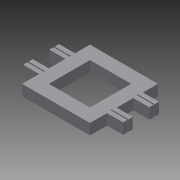
# Autodesk Inventor part: printed carriage v2
Saved by Autodesk Inventor 2014 SP1 (Build 180222100, 222)
## iProperties
Created: 2014-10-27
Part Number: printed carriage v2
Material: Generic
Document SubType Name: Modeling
Designer: dave
Density: 1 g/cm^3
Appearance: Default
Author: dave
Autodesk Inventor part; units mm, degrees
ref_plane "YZ Plane" through (0, 0, 0) normal (1, 0, 0) x (0, 1, 0)
ref_plane "XZ Plane" through (0, 0, 0) normal (0, 1, 0) x (-1, 0, 0)
ref_plane "XY Plane" through (0, 0, 0) normal (0, 0, 1) x (1, 0, 0)
sketch "Sketch1" plane through (0, 0, 0) normal (0, 0, 1) x (1, 0, 0)
  line L0 (0, 0) -> (63.5, 0)
  line L1 (63.5, 63.5) -> (0, 63.5)
  line L2 (0, 2) -> (0, 16) construction
  line L3 (0, 20.5) -> (-60, 20.5) construction
  line L4 (-60, 20.5) -> (152, 20.5) construction
  line L5 (0, 45) -> (-57, 45) construction
  line L6 (-57, 45) -> (114, 45) construction
  line L7 (0, 16) -> (-15, 16)
  line L8 (-15, 25) -> (0, 25)
  line L9 (0, 16) -> (0, 0)
  line L10 (0, 0) -> (12.5, 0) construction
  line L11 (12.5, 0) -> (12.5, 12.5) construction
  line L12 (12.5, 12.5) -> (18.4945, 12.5) construction
  line L13 (63.5, 63.5) -> (63.5, 51) construction
  line L14 (63.5, 51) -> (51, 51) construction
  line L15 (51, 51) -> (12.5, 51)
  line L16 (12.5, 51) -> (12.5, 12.5)
  line L17 (12.5, 12.5) -> (51, 12.5)
  line L18 (51, 12.5) -> (51, 51)
  line L19 (0, 40.5) -> (-15, 40.5)
  line L20 (-15, 49.5) -> (0, 49.5)
  line L21 (0.2886, 45.1642) -> (0.1212, 45.6242)
  line L22 (0.1212, 45.6242) -> (-0.6388, 45.6242)
  line L23 (-0.6388, 45.6242) -> (-0.8062, 45.1642)
  line L24 (-0.8062, 45.1642) -> (-1.7414, 45.1642)
  line L25 (-1.7414, 45.1642) -> (-1.9088, 45.6242)
  line L26 (-1.9088, 45.6242) -> (-2.6688, 45.6242)
  line L27 (-2.6688, 45.6242) -> (-2.8362, 45.1642)
  line L28 (-2.8362, 45.1642) -> (-3.7714, 45.1642)
  line L29 (-3.7714, 45.1642) -> (-3.9388, 45.6242)
  line L30 (-3.9388, 45.6242) -> (-4.6988, 45.6242)
  line L31 (-4.6988, 45.6242) -> (-4.8662, 45.1642)
  line L32 (-4.8662, 45.1642) -> (-5.8014, 45.1642)
  line L33 (-5.8014, 45.1642) -> (-5.9688, 45.6242)
  line L34 (-5.9688, 45.6242) -> (-6.7288, 45.6242)
  line L35 (-6.7288, 45.6242) -> (-6.8962, 45.1642)
  line L36 (-6.8962, 45.1642) -> (-7.8314, 45.1642)
  line L37 (-7.8314, 45.1642) -> (-7.9988, 45.6242)
  line L38 (-7.9988, 45.6242) -> (-8.7588, 45.6242)
  line L39 (-8.7588, 45.6242) -> (-8.9262, 45.1642)
  line L40 (-8.9262, 45.1642) -> (-9.8614, 45.1642)
  line L41 (-9.8614, 45.1642) -> (-10.0288, 45.6242)
  line L42 (-10.0288, 45.6242) -> (-10.7888, 45.6242)
  line L43 (-10.7888, 45.6242) -> (-10.9562, 45.1642)
  line L44 (-10.9562, 45.1642) -> (-11.8914, 45.1642)
  line L45 (-11.8914, 45.1642) -> (-12.0588, 45.6242)
  line L46 (-12.0588, 45.6242) -> (-12.8188, 45.6242)
  line L47 (-12.8188, 45.6242) -> (-12.9862, 45.1642)
  line L48 (-12.9862, 45.1642) -> (-13.9214, 45.1642)
  line L49 (-13.9214, 45.1642) -> (-14.0888, 45.6242)
  line L50 (-14.0888, 45.6242) -> (-14.8488, 45.6242)
  line L51 (-14.8488, 45.6242) -> (-15, 45.2088)
  line L52 (-15.0162, 44.4142) -> (0.2886, 44.4142)
  line L53 (0.3194, 20.653) -> (0.152, 21.113)
  line L54 (0.152, 21.113) -> (-0.608, 21.113)
  line L55 (-0.608, 21.113) -> (-0.7755, 20.653)
  line L56 (-0.7755, 20.653) -> (-1.7106, 20.653)
  line L57 (-1.7106, 20.653) -> (-1.878, 21.113)
  line L58 (-1.878, 21.113) -> (-2.638, 21.113)
  line L59 (-2.638, 21.113) -> (-2.8055, 20.653)
  line L60 (-2.8055, 20.653) -> (-3.7406, 20.653)
  line L61 (-3.7406, 20.653) -> (-3.908, 21.113)
  line L62 (-3.908, 21.113) -> (-4.668, 21.113)
  line L63 (-4.668, 21.113) -> (-4.8355, 20.653)
  line L64 (-4.8355, 20.653) -> (-5.7706, 20.653)
  line L65 (-5.7706, 20.653) -> (-5.938, 21.113)
  line L66 (-5.938, 21.113) -> (-6.698, 21.113)
  line L67 (-6.698, 21.113) -> (-6.8655, 20.653)
  line L68 (-6.8655, 20.653) -> (-7.8006, 20.653)
  line L69 (-7.8006, 20.653) -> (-7.968, 21.113)
  line L70 (-7.968, 21.113) -> (-8.728, 21.113)
  line L71 (-8.728, 21.113) -> (-8.8955, 20.653)
  line L72 (-8.8955, 20.653) -> (-9.8306, 20.653)
  line L73 (-9.8306, 20.653) -> (-9.998, 21.113)
  line L74 (-9.998, 21.113) -> (-10.758, 21.113)
  line L75 (-10.758, 21.113) -> (-10.9255, 20.653)
  line L76 (-10.9255, 20.653) -> (-11.8606, 20.653)
  line L77 (-11.8606, 20.653) -> (-12.028, 21.113)
  line L78 (-12.028, 21.113) -> (-12.788, 21.113)
  line L79 (-12.788, 21.113) -> (-12.9555, 20.653)
  line L80 (-12.9555, 20.653) -> (-13.8906, 20.653)
  line L81 (-13.8906, 20.653) -> (-14.058, 21.113)
  line L82 (-14.058, 21.113) -> (-14.8177, 21.113)
  line L83 (-14.8177, 21.113) -> (-15, 20.6122)
  line L84 (-15, 19.903) -> (0.3194, 19.903)
  line L85 (0, 63.5) -> (0, 49.5) construction
  line L86 (0, 63.5) -> (0, 49.5)
  line L87 (0, 40.5) -> (0, 25)
  line L88 (0.2886, 45.1642) -> (0.2886, 44.4142)
  line L89 (-15, 40.5) -> (-15, 44.4142)
  line L90 (-15, 45.2088) -> (-15, 49.5)
  line L91 (0.3194, 20.653) -> (0.3194, 19.903)
  line L92 (-15, 16) -> (-15, 19.903)
  line L93 (-15, 20.6122) -> (-15, 25)
  line L94 (63.5, 40.5) -> (78.5, 40.5)
  line L95 (78.5, 49.5) -> (63.5, 49.5)
  line L96 (63.5, 16) -> (78.5, 16)
  line L97 (63.5, 25) -> (78.5, 25)
  line L98 (78.5, 20.8487) -> (77.9976, 20.8487)
  line L99 (77.9976, 20.8487) -> (77.8302, 21.3087)
  line L100 (77.8302, 21.3087) -> (77.0702, 21.3087)
  line L101 (77.0702, 21.3087) -> (76.9027, 20.8487)
  line L102 (76.9027, 20.8487) -> (75.9676, 20.8487)
  line L103 (75.9676, 20.8487) -> (75.8002, 21.3087)
  line L104 (75.8002, 21.3087) -> (75.0402, 21.3087)
  line L105 (75.0402, 21.3087) -> (74.8727, 20.8487)
  line L106 (74.8727, 20.8487) -> (73.9376, 20.8487)
  line L107 (73.9376, 20.8487) -> (73.7702, 21.3087)
  line L108 (73.7702, 21.3087) -> (73.0102, 21.3087)
  line L109 (73.0102, 21.3087) -> (72.8427, 20.8487)
  line L110 (72.8427, 20.8487) -> (71.9076, 20.8487)
  line L111 (71.9076, 20.8487) -> (71.7402, 21.3087)
  line L112 (71.7402, 21.3087) -> (70.9802, 21.3087)
  line L113 (70.9802, 21.3087) -> (70.8127, 20.8487)
  line L114 (70.8127, 20.8487) -> (69.8776, 20.8487)
  line L115 (69.8776, 20.8487) -> (69.7102, 21.3087)
  line L116 (69.7102, 21.3087) -> (68.9502, 21.3087)
  line L117 (68.9502, 21.3087) -> (68.7827, 20.8487)
  line L118 (68.7827, 20.8487) -> (67.8476, 20.8487)
  line L119 (67.8476, 20.8487) -> (67.6802, 21.3087)
  line L120 (67.6802, 21.3087) -> (66.9202, 21.3087)
  line L121 (66.9202, 21.3087) -> (66.7527, 20.8487)
  line L122 (66.7527, 20.8487) -> (65.8176, 20.8487)
  line L123 (65.8176, 20.8487) -> (65.6502, 21.3087)
  line L124 (65.6502, 21.3087) -> (64.8902, 21.3087)
  line L125 (64.8902, 21.3087) -> (64.7227, 20.8487)
  line L126 (64.7227, 20.8487) -> (63.7876, 20.8487)
  line L127 (63.7876, 20.8487) -> (63.6202, 21.3087)
  line L128 (63.6202, 21.3087) -> (62.8602, 21.3087)
  line L129 (62.8602, 21.3087) -> (62.6927, 20.8487)
  line L130 (62.6927, 20.8487) -> (62.6927, 20.0987)
  line L131 (62.6927, 20.0987) -> (78.5, 20.0987)
  line L132 (78.5, 45.3158) -> (77.9976, 45.3158)
  line L133 (77.9976, 45.3158) -> (77.8302, 45.7758)
  line L134 (77.8302, 45.7758) -> (77.0702, 45.7758)
  line L135 (77.0702, 45.7758) -> (76.9027, 45.3158)
  line L136 (76.9027, 45.3158) -> (75.9676, 45.3158)
  line L137 (75.9676, 45.3158) -> (75.8002, 45.7758)
  line L138 (75.8002, 45.7758) -> (75.0402, 45.7758)
  line L139 (75.0402, 45.7758) -> (74.8727, 45.3158)
  line L140 (74.8727, 45.3158) -> (73.9376, 45.3158)
  line L141 (73.9376, 45.3158) -> (73.7702, 45.7758)
  line L142 (73.7702, 45.7758) -> (73.0102, 45.7758)
  line L143 (73.0102, 45.7758) -> (72.8427, 45.3158)
  line L144 (72.8427, 45.3158) -> (71.9076, 45.3158)
  line L145 (71.9076, 45.3158) -> (71.7402, 45.7758)
  line L146 (71.7402, 45.7758) -> (70.9802, 45.7758)
  line L147 (70.9802, 45.7758) -> (70.8127, 45.3158)
  line L148 (70.8127, 45.3158) -> (69.8776, 45.3158)
  line L149 (69.8776, 45.3158) -> (69.7102, 45.7758)
  line L150 (69.7102, 45.7758) -> (68.9502, 45.7758)
  line L151 (68.9502, 45.7758) -> (68.7827, 45.3158)
  line L152 (68.7827, 45.3158) -> (67.8476, 45.3158)
  line L153 (67.8476, 45.3158) -> (67.6802, 45.7758)
  line L154 (67.6802, 45.7758) -> (66.9202, 45.7758)
  line L155 (66.9202, 45.7758) -> (66.7527, 45.3158)
  line L156 (66.7527, 45.3158) -> (65.8176, 45.3158)
  line L157 (65.8176, 45.3158) -> (65.6502, 45.7758)
  line L158 (65.6502, 45.7758) -> (64.8902, 45.7758)
  line L159 (64.8902, 45.7758) -> (64.7227, 45.3158)
  line L160 (64.7227, 45.3158) -> (63.7876, 45.3158)
  line L161 (63.7876, 45.3158) -> (63.6202, 45.7758)
  line L162 (63.6202, 45.7758) -> (62.8602, 45.7758)
  line L163 (62.8602, 45.7758) -> (62.6927, 45.3158)
  line L164 (62.6927, 45.3158) -> (62.6927, 44.5658)
  line L165 (62.6927, 44.5658) -> (78.5, 44.5658)
  line L166 (78.5, 16) -> (78.5, 20.0987)
  line L167 (78.5, 20.8487) -> (78.5, 25)
  line L168 (63.5, 0) -> (63.5, 16)
  line L169 (63.5, 49.5) -> (63.5, 63.5)
  line L170 (63.5, 25) -> (63.5, 40.5)
  line L171 (78.5, 40.5) -> (78.5, 44.5658)
  line L172 (78.5, 45.3158) -> (78.5, 49.5)
  dimension "d0" = 63.5
  dimension "d5" = 16
  dimension "d6" = 12.5
  dimension "d7" = 12.5
  dimension "d8" = 12.5
  dimension "d9" = 12.5
  dimension "d11" = 15
  dimension "d12" = 9
  constraints: 346 end point, 30 perpendicular, 21 parallel, 7 point on line, 2 horizontal
  measures "d0" distance of L1.end L1.start
  measures "d5" distance of L2.end L0.start
  measures "d6" distance of L0.start L10.end
  measures "d7" distance of L10.end L11.end
  measures "d8" distance of L1.start L13.end
  measures "d9" distance of L13.end L14.end
  measures "d11" distance of L19.start L19.end
  measures "d12" distance of L19.end L20.start
extrude "Extrusion1" add sketch "Sketch1" along normal blind 10
body "Solid1"
